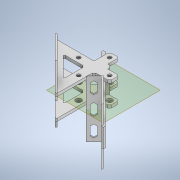
# Autodesk Inventor part: Holder_v2
Saved by Autodesk Inventor 2020 (Build 240168000, 168)
## iProperties
Created: 2019-12-20
Part Number: Holder_v2
Material: Generic
Document SubType Name: Modeling
Designer: atmat
Density: 1 g/cm^3
Appearance: Default
Author: atmat
Autodesk Inventor part; units mm, degrees
ref_plane "YZ Plane" through (0, 0, 0) normal (1, 0, 0) x (0, 1, 0)
ref_plane "XZ Plane" through (0, 0, 0) normal (0, 1, 0) x (-1, 0, 0)
ref_plane "XY Plane" through (0, 0, 0) normal (0, 0, 1) x (1, 0, 0)
sketch "Sketch1" plane through (0, 0, 0) normal (0, 1, 0) x (-1, 0, 0)
  circle A0 centre (0, 16.5) radius 2
  circle A1 centre (0, -16.5) radius 2
  circle A2 centre (16.5, 0) radius 2
  circle A3 centre (-16.5, 0) radius 2
  line L0 (5, 21.5) -> (-5, 21.5)
  line L1 (-5, 21.5) -> (-5, -21.5)
  line L2 (-5, -21.5) -> (5, -21.5)
  line L3 (5, -21.5) -> (5, 21.5)
  line L4 (21.5, 5) -> (-21.5, 5)
  line L5 (-21.5, 5) -> (-21.5, -5)
  line L6 (-21.5, -5) -> (21.5, -5)
  line L7 (21.5, -5) -> (21.5, 5)
  point P0 (0, 0)
  point P1 (-5, 5)
  point P2 (-5, -5)
  point P3 (5, -5)
  point P4 (5, 5)
  dimension "d0" = 4
  dimension "d1" = 4
  dimension "d2" = 16.5
  dimension "d3" = 16.5
  dimension "d4" = 4
  dimension "d5" = 4
  dimension "d6" = 16.5
  dimension "d7" = 16.5
  dimension "d8" = 3
  dimension "d9" = 10
  dimension "d10" = 3
  dimension "d11" = 3
  dimension "d12" = 5
  dimension "d13" = 5
  dimension "d14" = 5
  dimension "d15" = 5
  constraints: 16 end point, 4 centre point, 4 parallel, 2 horizontal, 2 perpendicular
  measures "d0" diameter of A0
  measures "d1" diameter of A1
  measures "d2" distance of point (0, 0) A0.centre
  measures "d3" distance of point (0, 0) A1.centre
  measures "d4" diameter of A2
  measures "d5" diameter of A3
  measures "d6" distance of point (0, 0) A2.centre
  measures "d7" distance of point (0, 0) A3.centre
  measures "d8" distance edge to line of A0 L3
  measures "d9" distance between parallel lines of L3 L1
  measures "d10" distance edge to line of A0 L0
  measures "d11" distance edge to line of A1 L2
  measures "d12" distance from line of L4 A2.centre
  measures "d13" distance from line of A2.centre L6
  measures "d14" distance from line of A2.centre L7
  measures "d15" distance from line of A3.centre L5
extrude "Extrusion1" add sketch "Sketch1" along normal blind 3
chamfer "Chamfer1" distance 2 angle 45 12 edges at (5, 1.5, -21.5) (21.5, 1.5, -5) (21.5, 1.5, 5) (-5, 1.5, -21.5) (5, 1.5, -5) (-5, 1.5, -5) (-21.5, 1.5, -5) (-21.5, 1.5, 5) (-5, 1.5, 21.5) (-5, 1.5, 5) (5, 1.5, 21.5) (5, 1.5, 5)
sketch "Sketch3" plane through (0, 0, 0) normal (0, -1, 0) x (1, 0, 0)
  line L0 (-11.6777, -23.6777) -> (59.033, 47.033)
  line L1 (59.033, 47.033) -> (56.9117, 49.1543)
  line L2 (56.9117, 49.1543) -> (-13.799, -21.5563)
  line L3 (-7, 5) -> (-5, 7) projected
  line L4 (7, -5) -> (5, -7) projected
  line L5 (5, 7) -> (7, 5) projected
  line L6 (-5, -7) -> (-7, -5) projected
  line L7 (-11.6777, -23.6777) -> (-13.799, -21.5563)
  point P0 (0, 0)
  dimension "d25" = 0
  dimension "d26" = 3
  dimension "d27" = 25
  dimension "d28" = 75
  constraints: 8 end point, 3 parallel, 1 collinear
  measures "d25" distance between parallel lines of L4 L0
  measures "d26" distance between parallel lines of L0 L2
  measures "d27" distance from line of L7 point (0, 0)
  measures "d28" distance from line of point (0, 0) L1
extrude "Extrusion2" add sketch "Sketch3" along normal blind 10
ref_plane "Work Plane1" through (0, -10, 0) normal (0, -1, 0) x (1, 0, 0)
mirror "Mirror1" about plane through (0, -10, 0) normal (0, -1, 0) of "Extrusion1", "Chamfer1", "Extrusion2"
chamfer "Chamfer2" distance 1.5 angle 45 4 edges at (59.033, -10, 47.033) (56.9117, -10, 49.1543) (-11.6777, -10, -23.6777) (-13.799, -10, -21.5563)
sketch "Sketch4" plane through (5, 0, -7) normal (0.7071068, 0, -0.7071068) x (-0.7071068, 0, -0.7071068)
  line L0 (-11.6673, 3) -> (-2.8284, 3) projected
  line L1 (8.8388, -23) -> (0, -23) projected
  line L2 (-6.4142, 3) -> (3.5858, 3)
  line L3 (3.5858, 3) -> (3.5858, -23)
  line L4 (3.5858, -23) -> (-6.4142, -23)
  line L5 (-6.4142, -23) -> (-6.4142, 3)
  point P0 (-1.4142, 0)
  point P1 (0, -23)
  point P2 (-2.8284, 3)
  dimension "d35" = 5
  dimension "d36" = 5
  constraints: 8 end point, 2 parallel, 2 point on line, 1 horizontal, 1 perpendicular
  measures "d35" distance from line of point (-1.414, 0) L5
  measures "d36" distance from line of L3 point (-1.414, 0)
extrude "Extrusion3" add sketch "Sketch4" along normal blind 3
chamfer "Chamfer3" distance 3 angle 45 2 edges at (4.5858, -10, -11.6569) (11.6569, -10, -4.5858)
sketch "Sketch5" plane through (-19.5, -20, -5) normal (0, 1, 0) x (1, 0, 0)
  line L0 (12.5, 0) -> (0, 0) projected
  line L1 (0, 0) -> (-26.9706, 0)
  line L2 (-26.9706, 0) -> (24.5, -51.4706)
  line L3 (24.5, -24.5) -> (24.5, -12) projected
  line L4 (24.5, -51.4706) -> (24.5, -24.5)
  line L5 (16.5, -26.5) -> (22.5, -26.5) projected
  line L6 (24.5, -24.5) -> (22.5, -26.5)
  line L7 (22.5, -26.5) -> (16.5, -26.5)
  line L8 (16.5, -26.5) -> (14.5, -24.5) projected
  line L9 (16.5, -26.5) -> (14.5, -24.5)
  line L10 (14.5, -12) -> (12.5, -10) projected
  line L11 (-2, -8) -> (0, -10) projected
  line L12 (0, -10) -> (-2, -8)
  line L13 (-2, -2) -> (-2, -8) projected
  line L14 (-2, -8) -> (-2, -2)
  line L15 (0, 0) -> (-2, -2) projected
  line L16 (-2, -2) -> (0, 0)
  line L17 (0, -10) -> (12.5, -10) projected
  line L18 (14.5, -12) -> (14.5, -24.5) projected
  line L19 (0, -10) -> (-8.4853, -10)
  line L20 (-8.4853, -10) -> (14.5, -32.9853)
  line L21 (14.5, -32.9853) -> (14.5, -24.5)
  line L22 (0, -10) -> (12.5, -10) projected
  point P0 (19.5, -5)
  dimension "d42" = 6
  dimension "d43" = 6
  constraints: 24 end point, 7 collinear, 3 parallel, 2 perpendicular, 1 horizontal
  measures "d42" distance between parallel lines of L20 L2
  measures "d43" distance between parallel lines of L12 L20
extrude "Extrusion4" add sketch "Sketch5" against normal blind 3 contours L15 L13 L11 L19 L20 L21 L8 L5 L6 L4 L2 L1
chamfer "Chamfer4" distance 2 angle 45 4 edges at (5, -21.5, 46.4706) (-46.4706, -21.5, -5) (-27.9853, -21.5, 5) (-5, -21.5, 27.9853)
sketch "Sketch6" plane through (7, -20, 5) normal (0, 1, 0) x (1, 0, 0)
  circle A0 centre (-23.5, 5) radius 3
  circle A1 centre (-23.5, 5) radius 2 projected
  circle A2 centre (-7, -11.5) radius 2 projected
  circle A3 centre (-7, -11.5) radius 3
  circle A4 centre (9.5, 5) radius 2 projected
  circle A5 centre (9.5, 5) radius 3
  circle A6 centre (-7, 21.5) radius 3
  circle A7 centre (-7, 21.5) radius 2 projected
  circle A8 centre (9.5, 5) radius 2 projected
  point P0 (-7, 5)
  dimension "d50" = 6
  dimension "d51" = 6
  dimension "d54" = 6
  dimension "d55" = 6
  constraints: 4 centre point, 3 concentric, 2 coincident
  measures "d50" diameter of A0
  measures "d51" diameter of A3
  measures "d54" diameter of A5
  measures "d55" diameter of A6
extrude "Extrusion5" cut sketch "Sketch6" against normal blind 2
sketch "Sketch7" plane through (7, -23, 5) normal (0, -1, 0) x (1, 0, 0)
  line L0 (-52.0563, -8.5858) -> (-3.4142, 40.0563) projected
  line L1 (-51.4706, -10) -> (-14, -10) projected
  line L2 (-52.0563, -8.5858) -> (-51.4706, -10)
  line L3 (-2, 39.4706) -> (-2, 2) projected
  line L4 (-51.4706, -10) -> (-2, 39.4706)
  line L5 (-2, 39.4706) -> (-3.4142, 40.0563)
  line L6 (-52.0563, -8.5858) -> (-3.4142, 40.0563)
  point P0 (-7, -5)
  constraints: 8 end point, 1 collinear
extrude "Extrusion6" add sketch "Sketch7" along normal blind 18
sketch "Sketch8" plane through (5, -41, 44.4706) normal (0.7071068, 0, -0.7071068) x (-0.7071068, 0, -0.7071068)
  line L0 (0, 18) -> (69.9619, 18) projected
  line L1 (69.9619, 18) -> (51.9619, 0)
  line L2 (0.5858, 0) -> (69.3762, 0) projected
  line L3 (69.9619, 18) -> (69.9619, 0) projected
  line L4 (69.3762, 0) -> (69.9619, 0) projected
  line L5 (69.9619, 18) -> (69.9619, 0)
  line L6 (69.9619, 0) -> (51.9619, 0)
  line L7 (0, 18) -> (26.4957, 18) projected
  line L8 (0, 18) -> (18, 0)
  line L9 (0, 0) -> (0.5858, 0) projected
  line L10 (18, 0) -> (0, 0)
  line L11 (0, 18) -> (0, 21) projected
  line L12 (0, 0) -> (0, 18)
  line L13 (46.4767, 3) -> (58.4767, 15)
  line L14 (58.4767, 15) -> (11.4853, 15)
  line L15 (11.4853, 15) -> (23.4853, 3)
  line L16 (23.4853, 3) -> (46.4767, 3)
  line L17 (69.9619, 0) -> (0, 0) projected
  line L18 (26.4853, 15) -> (38.4853, 3)
  line L19 (30.7279, 15) -> (42.7279, 3)
  line L20 (27.234, 3) -> (39.234, 15)
  line L21 (43.4767, 15) -> (31.4767, 3)
  point P0 (34.981, 41)
  point P1 (18, 0)
  point P2 (37.1023, 8.6256)
  point P3 (34.981, 10.747)
  point P4 (34.981, 6.5043)
  point P5 (32.8597, 8.6256)
  dimension "d58" = 45
  dimension "d59" = 45
  dimension "d60" = 3
  dimension "d61" = 3
  dimension "d62" = 6
  dimension "d63" = 6
  dimension "d80" = 3
  dimension "d81" = 3
  dimension "d82" = 15
  dimension "d83" = 15
  constraints: 28 end point, 10 point on line, 7 parallel, 2 collinear, 2 perpendicular, 1 horizontal, 1 vertical
  measures "d58" angle of L3 L1
  measures "d59" angle of L8 L12
  measures "d60" distance between parallel lines of L2 L16
  measures "d61" distance between parallel lines of L0 L14
  measures "d62" distance between parallel lines of L1 L13
  measures "d63" distance between parallel lines of L8 L15
  measures "d80" distance between parallel lines of L19 L18
  measures "d81" distance between parallel lines of L20 L21
  measures "d82" distance of L14.end L18.start
  measures "d83" distance of L13.end L21.start
extrude "Extrusion7" cut sketch "Sketch8" against normal blind 2 contours L8 L2 L9 L12 | L3 L4 L2 L1 | L16 L19 L21 L14 L13 | L16 L21 L18 | L20 L19 L14 | L16 L15 L14 L18 L20
mirror "Mirror5" about plane through (0, -10, 0) normal (0, -1, 0) of "Extrusion4"
mirror "Mirror6" about plane through (0, -10, 0) normal (0, -1, 0) of "Extrusion5", "Extrusion6", "Extrusion7"
chamfer "Chamfer5" distance 2 angle 45 4 edges at (-46.4706, 1.5, -5) (5, 1.5, 46.4706) (-27.9853, 1.5, 5) (-5, 1.5, 27.9853)
sketch "Sketch9" plane through (0, -10, 0) normal (0, -1, 0) x (1, 0, 0)
  line L0 (55.851, 48.0937) -> (12.7574, 5) projected
  line L1 (30.3952, 22.6378) -> (22.2635, 30.7696)
  line L2 (55.851, 48.0937) -> (12.7574, 5) projected
  line L3 (57.9723, 48.0937) -> (55.851, 48.0937) projected
  line L4 (57.9723, 45.9723) -> (57.9723, 48.0937) projected
  line L5 (55.851, 48.0937) -> (57.9723, 45.9723)
  line L6 (22.2635, 30.7696) -> (21.2028, 29.7089)
  line L7 (21.2028, 29.7089) -> (29.3345, 21.5772)
  line L8 (30.3952, 22.6378) -> (29.3345, 21.5772)
  line L9 (30.3952, 22.6378) -> (55.851, 48.0937)
  line L10 (29.3345, 21.5772) -> (30.3952, 20.5165)
  line L11 (30.3952, 20.5165) -> (56.9117, 47.033)
  point P0 (0, 0)
  dimension "d69" = 36
  dimension "d70" = 11.5
  dimension "d71" = 1.5
  constraints: 16 end point, 3 point on line, 2 collinear, 2 perpendicular, 1 midpoint, 1 parallel
  measures "d69" distance between parallel lines of L1 L5
  measures "d70" distance of L1.start L1.end
  measures "d71" distance between parallel lines of L7 L1
extrude "Extrusion8" add sketch "Sketch9" against normal mid plane 60 contours L5 L11 L10 L0 | L0 L7 L6 L1
chamfer "Chamfer6" distance 1.5 angle 45 3 edges at (56.9117, -30, 47.033) (56.9117, 10, 47.033) (21.2028, -10, 29.7089)
sketch "Sketch10" plane through (57.9723, -20, 45.9723) normal (0.7071068, 0, -0.7071068) x (-0.7071068, 0, -0.7071068)
  line L0 (8.5173, 7) -> (26.5173, 7)
  line L1 (26.5173, 7) -> (29.0346, 10)
  line L2 (29.0346, 10) -> (26.5173, 13)
  line L3 (26.5173, 13) -> (8.5173, 13)
  line L4 (8.5173, 13) -> (6, 10)
  line L5 (6, 10) -> (8.5173, 7)
  line L6 (57.9437, 0) -> (0, 0) projected
  line L7 (57.9437, 20) -> (0, 20) projected
  line L8 (0, 0) -> (0, 20) projected
  point P0 (73.5, 20)
  dimension "d87" = 130
  dimension "d88" = 3
  dimension "d89" = 6
  dimension "d90" = 10
  dimension "d91" = 6
  dimension "d92" = 0
  dimension "d93" = 0
  dimension "d94" = 18
  constraints: 12 end point, 4 parallel, 1 horizontal
  measures "d87" angle of L0 L1
  measures "d88" distance from line of L0 L4.end
  measures "d89" distance between parallel lines of L0 L3
  measures "d90" distance from line of L6 L4.end
  measures "d91" distance from line of L8 L4.end
  measures "d92" horizontal distance of L3.end L0.start
  measures "d93" horizontal distance of L0.end L2.end
  measures "d94" distance of L2.end L3.end
extrude "Extrusion9" cut sketch "Sketch10" against normal blind 3
mirror "Mirror7" about plane through (22.617, -20, 12.7383) normal (0, -1, 0) of "Extrusion9"
mirror "Mirror8" about plane through (22.617, 0, 12.7383) normal (0, 1, 0) of "Extrusion9"
sketch "Sketch11" plane through (3.5858, 0, 45.0563) normal (-0.7071068, 0, 0.7071068) x (0.7071068, 0, 0.7071068)
  line L0 (-68.7904, 0) -> (0, 0) projected
  line L1 (-46.5164, 0) -> (-26.5164, -20)
  line L2 (-68.7904, -20) -> (0, -20) projected
  line L3 (-22.2737, -20) -> (-42.2737, 0)
  line L4 (-42.2737, 0) -> (-46.5164, 0)
  line L5 (-26.5164, -20) -> (-22.2737, -20)
  line L6 (-26.5164, 0) -> (-46.5164, -20)
  line L7 (-46.5164, -20) -> (-42.2737, -20)
  line L8 (-42.2737, -20) -> (-22.2737, 0)
  line L9 (-26.5164, 0) -> (-22.2737, 0)
  line L10 (-38.6482, 6) -> (-34.3952, 10.253) projected
  line L11 (-34.3952, 10.253) -> (-30.1421, 6) projected
  point P0 (-34.3952, 0)
  point P1 (-34.395, -7.8787)
  point P2 (-42.2737, 0)
  point P3 (-36.5164, -10)
  point P4 (-34.395, -12.1213)
  point P5 (-22.2737, -20)
  point P6 (-32.2737, -10)
  dimension "d97" = 3
  dimension "d98" = 3
  dimension "d101" = 22.274
  dimension "d102" = 22.274
  constraints: 16 end point, 9 point on line, 5 parallel, 1 collinear, 1 horizontal
  measures "d97" distance between parallel lines of L3 L1
  measures "d98" distance between parallel lines of L6 L8
  measures "d101" distance of L1.start L0.start
  measures "d102" distance of L2.start L6.end
extrude "Extrusion10" add sketch "Sketch11" against normal blind 1.414 contours L0 L3 L6 L1 | L6 L3 L8 L1 | L1 L8 L2 L6 | L0 L8 L3 L6 | L8 L3 L2 L1
sketch "Sketch12" plane through (30.3952, -40, 22.6378) normal (0.7071068, 0, 0.7071068) x (0.7071068, 0, -0.7071068)
  line L0 (-8.5, 34.5) -> (-8.5, 25.5)
  line L1 (-8.5, 25.5) -> (-5.75, 23.6499)
  line L2 (-5.75, 23.6499) -> (-3, 25.5)
  line L3 (-3, 25.5) -> (-3, 34.5)
  line L4 (-3, 34.5) -> (-5.75, 36.3501)
  line L5 (-5.75, 36.3501) -> (-8.5, 34.5)
  line L6 (-11.5, 0) -> (-11.5, 60) projected
  line L7 (0, 40) -> (0, 20) projected
  line L8 (76.0705, 30) -> (-95.9227, 30) projected
  point P0 (-5.4853, 40)
  dimension "d105" = 0
  dimension "d106" = 3
  dimension "d107" = 3
  dimension "d108" = 2.75
  dimension "d109" = 0
  dimension "d110" = 9
  dimension "d112" = 4.5
  constraints: 12 end point, 4 parallel, 1 vertical
  measures "d105" vertical distance of L2.end L0.end
  measures "d106" distance between parallel lines of L6 L0
  measures "d107" distance between parallel lines of L7 L3
  measures "d108" distance from line of L0 L4.end
  measures "d109" vertical distance of L0.start L3.end
  measures "d110" distance of L2.end L3.end
  measures "d112" distance from line of L3.end L8
extrude "Extrusion11" cut sketch "Sketch12" against normal blind 1.5
mirror "Mirror9" about plane through (22.617, 0, 12.7383) normal (0, 1, 0) of "Extrusion11"
mirror "Mirror10" about plane through (22.617, -20, 12.7383) normal (0, -1, 0) of "Extrusion11"
body "Solid1"
